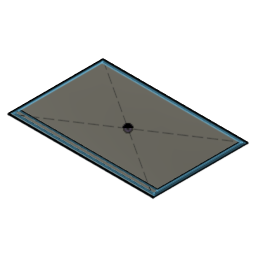
ecran (Autodesk Fusion 360 design; units mm, degrees)
Autodesk Fusion 360 part; units mm, degrees
sketch "Sketch1" plane through (0, 0, 0) normal (0, 0, 1) x (1, 0, 0)
  line L0 (-85.1, 55.6) -> (85.1, 55.6)
  line L1 (85.1, 55.6) -> (85.1, -55.6)
  line L2 (85.1, -55.6) -> (-85.1, -55.6)
  line L3 (-85.1, -55.6) -> (-85.1, 55.6)
  line L4 (-85.1, 55.6) -> (85.1, -55.6) construction
  line L5 (85.1, 55.6) -> (-85.1, -55.6) construction
  line L6 (-84.0199, 54.3533) -> (83.7801, 54.3533)
  line L7 (83.7801, 54.3533) -> (83.7801, -52.7367)
  line L8 (83.7801, -52.7367) -> (-84.0199, -52.7367)
  line L9 (-84.0199, -52.7367) -> (-84.0199, 54.3533)
  line L10 (-83.0921, 52.8533) -> (81.7079, 52.8533)
  line L11 (81.7079, 52.8533) -> (81.7079, -51.2367)
  line L12 (81.7079, -51.2367) -> (-83.0921, -51.2367)
  line L13 (-83.0921, -51.2367) -> (-83.0921, 52.8533)
  line L14 (-82.6768, 52.0533) -> (80.5232, 52.0533)
  line L15 (80.5232, 52.0533) -> (80.5232, -45.8667)
  line L16 (-82.6768, 52.0533) -> (-82.6768, -45.8667)
  line L17 (-82.6768, -45.8667) -> (80.5232, -45.8667)
  dimension "d1" = 170.2
  dimension "d2" = 111.2
  dimension "d5" = 107.09
  dimension "d9" = 164.8
  dimension "d10" = 104.09
  dimension "d12" = 163.2
  dimension "d14" = 97.92
  constraint horizontal L0
  constraint perpendicular L0 L1
  constraint parallel L0 L2
  constraint parallel L1 L3
  constraint coincident L4 origin
  constraint coincident L5 origin
  constraint horizontal L6
  constraint vertical L7
  constraint horizontal L8
  constraint vertical L9
  constraint horizontal L10
  constraint vertical L11
  constraint horizontal L12
  constraint vertical L13
  constraint horizontal L14
  constraint perpendicular L14 L15
  constraint perpendicular L15 L17
  measures "d1" distance of L1.end L2.end
  measures "d2" distance of L0.end L1.end
  measures "d5" distance of L6.start L8.end
  measures "d9" distance of L10.start L10.end
  measures "d10" distance of L10.start L12.end
  measures "d12" distance of L14.start L14.end
  measures "d14" distance of L14.end L15.end
extrude "Extrude1" add sketch "Sketch1" along normal blind 0.7 contours L0 L1 L2 L3
extrude "Extrude2" add sketch "Sketch1" along normal blind 0.13 contours L6 L7 L8 L9
extrude "Extrude3" add sketch "Sketch1" along normal blind 0.07 contours L10 L11 L12 L13
extrude "Extrude4" add sketch "Sketch1" along normal blind 1.18 contours L14 L15 L16 L17
